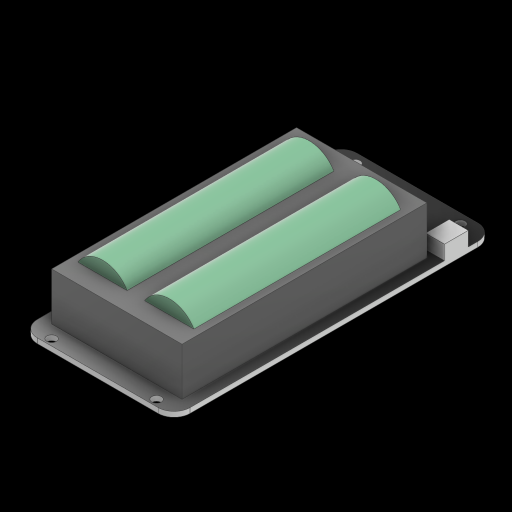
# Autodesk Inventor part: 010_Battery_2Cell
Saved by Autodesk Inventor 2024 (Build 280153000, 153)
## iProperties
Created: 2023-07-20
Part Number: 010_Battery_2Cell
Material: Generisch
Document SubType Name: Modeling
Designer: Philipp
Density: 1 g/cm^3
Appearance: Vorgabe
Author: Philipp
Autodesk Inventor part; units mm, degrees
ref_plane "YZ Plane" through (0, 0, 0) normal (1, 0, 0) x (0, 1, 0)
ref_plane "XZ Plane" through (0, 0, 0) normal (0, 1, 0) x (-1, 0, 0)
ref_plane "XY Plane" through (0, 0, 0) normal (0, 0, 1) x (1, 0, 0)
sketch "Skizze1" plane through (0, 0, 0) normal (0, 0, 1) x (1, 0, 0)
  line L0 (24, 50.25) -> (-24, 50.25)
  line L1 (-24, 50.25) -> (-24, -50.25)
  line L2 (-24, -50.25) -> (24, -50.25)
  line L3 (24, -50.25) -> (24, 50.25)
  line L4 (24, 50.25) -> (-24, -50.25) construction
  line L5 (-24, 50.25) -> (24, -50.25) construction
  point P0 (0, 0)
  dimension "d0" = 48
  dimension "d1" = 100.5
  constraints: 12 end point, 2 midpoint, 2 parallel, 1 horizontal, 1 perpendicular
  measures "d0" distance of L2.end L1.end
  measures "d1" distance of L1.end L0.end
extrude "Extrusion1" add sketch "Skizze1" along normal blind 1.6
fillet "Rundung1" radius 5 4 edges at (24, 50.25, 0.8) (-24, 50.25, 0.8) (24, -50.25, 0.8) (-24, -50.25, 0.8)
sketch "Skizze2" plane through (0, 0, 0) normal (0, 0, -1) x (-1, 0, 0)
  line L0 (-6.5, -11.25) -> (0, -11.25)
  line L1 (0, -11.25) -> (0, -17.75)
  line L2 (0, -17.75) -> (-6.5, -17.75)
  line L3 (-6.5, -17.75) -> (-6.5, -11.25)
  line L4 (-6.5, -11.25) -> (0, -17.75) construction
  line L5 (0, -11.25) -> (-6.5, -17.75) construction
  line L6 (19, -50.25) -> (-19, -50.25) projected
  line L7 (-24, -45.25) -> (-24, 45.25) projected
  point P0 (0, 0)
  point P1 (-3.25, -14.5)
  point P2 (-3.25, -17.75)
  dimension "d5" = 32.5
  dimension "d6" = 17.5
  dimension "d7" = 6.5
  dimension "d8" = 6.5
  constraints: 12 end point, 3 midpoint, 2 parallel, 1 horizontal, 1 perpendicular
  measures "d5" distance from line of L6 point (-3.25, -17.75)
  measures "d6" distance between parallel lines of L7 L3
  measures "d7" distance of L2.end L0.start
  measures "d8" distance of L0.start L0.end
extrude "Extrusion2" add sketch "Skizze2" along normal blind 5
fillet "Rundung2" radius 0.5 4 edges at (0, -11.25, -2.5) (0, -17.75, -2.5) (6.5, -17.75, -2.5) (6.5, -11.25, -2.5)
sketch "Skizze3" plane through (0, 0, 0) normal (0, 0, -1) x (-1, 0, 0)
  line L0 (17, -33.75) -> (24, -33.75)
  line L1 (24, -33.75) -> (24, -42.75)
  line L2 (24, -42.75) -> (17, -42.75)
  line L3 (17, -42.75) -> (17, -33.75)
  line L4 (17, -33.75) -> (24, -42.75) construction
  line L5 (24, -33.75) -> (17, -42.75) construction
  line L6 (19, -50.25) -> (-19, -50.25) projected
  line L7 (24, 45.25) -> (24, -45.25) projected
  point P0 (0, 0)
  point P1 (20.5, -38.25)
  dimension "d12" = 7.5
  dimension "d13" = 7
  dimension "d14" = 9
  constraints: 12 end point, 2 midpoint, 2 parallel, 1 collinear, 1 horizontal, 1 perpendicular
  measures "d12" distance between parallel lines of L6 L2
  measures "d13" distance of L1.end L2.end
  measures "d14" distance of L2.end L0.start
extrude "Extrusion3" add sketch "Skizze3" along normal blind 5
fillet "Rundung3" radius 2 2 edges at (-20.5, -33.75, -5) (-20.5, -42.75, -5)
sketch "Skizze4" plane through (0, 0, 1.6) normal (0, 0, 1) x (1, 0, 0)
  line L0 (18, 42.25) -> (24, 42.25)
  line L1 (24, 42.25) -> (24, 34.75)
  line L2 (24, 34.75) -> (18, 34.75)
  line L3 (18, 34.75) -> (18, 42.25)
  line L4 (18, 42.25) -> (24, 34.75) construction
  line L5 (24, 42.25) -> (18, 34.75) construction
  line L6 (24, -45.25) -> (24, 45.25) projected
  line L7 (-24, 45.25) -> (-24, -45.25) projected
  line L8 (19, 50.25) -> (-19, 50.25) projected
  line L9 (-22, 42.25) -> (-17.5, 42.25)
  line L10 (-17.5, 42.25) -> (-17.5, 33.25)
  line L11 (-17.5, 33.25) -> (-22, 33.25)
  line L12 (-22, 33.25) -> (-22, 42.25)
  line L13 (-22, 42.25) -> (-17.5, 33.25) construction
  line L14 (-17.5, 42.25) -> (-22, 33.25) construction
  point P0 (0, 0)
  point P1 (21, 38.5)
  point P2 (21, 42.25)
  point P3 (-19.75, 37.75)
  dimension "d19" = 8
  dimension "d20" = 7.5
  dimension "d21" = 6
  dimension "d22" = 8
  dimension "d23" = 9
  dimension "d24" = 4.5
  dimension "d25" = 2
  constraints: 24 end point, 5 midpoint, 4 parallel, 2 horizontal, 2 perpendicular, 1 collinear
  measures "d19" distance from line of L8 point (21, 42.25)
  measures "d20" distance of L2.end L0.start
  measures "d21" distance of L1.end L2.end
  measures "d22" distance between parallel lines of L8 L9
  measures "d23" distance of L9.end L10.end
  measures "d24" distance of L10.end L11.end
  measures "d25" distance between parallel lines of L7 L12
extrude "Extrusion4" add sketch "Skizze4" along normal blind 4.5
sketch "Skizze5" plane through (-22, 33.25, 1.6) normal (-1, 0, 0) x (0, 0, 1)
  line L0 (1.5, 1.5) -> (3.5, 1.5)
  line L1 (3.5, 1.5) -> (3.5, 7.5)
  line L2 (3.5, 7.5) -> (1.5, 7.5)
  line L3 (1.5, 7.5) -> (1.5, 1.5)
  line L4 (1.5, 1.5) -> (3.5, 7.5) construction
  line L5 (3.5, 1.5) -> (1.5, 7.5) construction
  line L6 (0, 9) -> (4.5, 9) projected
  line L7 (4.5, 9) -> (4.5, 0) projected
  point P0 (-1.6, -33.25)
  point P1 (2.5, 4.5)
  dimension "d28" = 1.5
  dimension "d29" = 6
  dimension "d30" = 1
  dimension "d31" = 2
  constraints: 12 end point, 2 midpoint, 2 parallel, 1 horizontal, 1 perpendicular
  measures "d28" distance between parallel lines of L6 L2
  measures "d29" distance of L0.end L1.end
  measures "d30" distance between parallel lines of L7 L1
  measures "d31" distance of L1.end L2.end
extrude "Extrusion5" add sketch "Skizze5" along normal blind 3
sketch "Skizze6" plane through (0, 0, 1.6) normal (0, 0, 1) x (1, 0, 0)
  line L0 (-20.5, 32.75) -> (20.5, 32.75)
  line L1 (20.5, 32.75) -> (20.5, -44.25)
  line L2 (20.5, -44.25) -> (-20.5, -44.25)
  line L3 (-20.5, -44.25) -> (-20.5, 32.75)
  line L4 (-20.5, 32.75) -> (20.5, -44.25) construction
  line L5 (20.5, 32.75) -> (-20.5, -44.25) construction
  line L6 (-19, -50.25) -> (19, -50.25) projected
  line L7 (24, -45.25) -> (24, 34.75) projected
  line L8 (-24, 45.25) -> (-24, -45.25) projected
  point P0 (0, 0)
  point P1 (0, -5.75)
  dimension "d34" = 6
  dimension "d35" = 3.5
  dimension "d36" = 3.5
  dimension "d37" = 77
  constraints: 12 end point, 2 midpoint, 2 parallel, 1 horizontal, 1 perpendicular
  measures "d34" distance between parallel lines of L6 L2
  measures "d35" distance between parallel lines of L7 L1
  measures "d36" distance between parallel lines of L8 L3
  measures "d37" distance of L2.end L0.start
extrude "Extrusion6" add sketch "Skizze6" along normal blind 15
sketch "Skizze7" plane through (-20.5, -44.25, 1.6) normal (0, -1, 0) x (1, 0, 0)
  circle A0 centre (10, 10.4) radius 9
  circle A1 centre (31, 10.4) radius 9
  line L0 (1.5, -1.6) -> (39.5, -1.6) projected
  line L1 (1.5, 0) -> (39.5, 0) projected
  point P0 (20.5, -1.6)
  point P1 (20.5, 0)
  dimension "d40" = 18
  dimension "d41" = 18
  dimension "d42" = 21
  dimension "d43" = 21
  dimension "d44" = 21
  dimension "d45" = 10.5
  constraints: 2 centre point, 1 midpoint
  measures "d40" diameter of A1
  measures "d41" diameter of A0
  measures "d44" distance of A1.centre A0.centre
  measures "d45" horizontal distance of point (20.5, 0) A0.centre
extrude "Extrusion7" add sketch "Skizze7" against normal blind 77
sketch "Skizze8" plane through (0, 0, 16.6) normal (0, 0, 1) x (1, 0, 0)
  line L0 (-18.2356, -44.25) -> (-18.2356, 32.75) projected
  line L1 (-18.2356, 32.75) -> (-20.5, 32.75) projected
  line L2 (-20.5, 32.75) -> (-20.5, -44.25) projected
  line L3 (-20.5, -44.25) -> (-18.2356, -44.25) projected
  line L4 (18.2356, 32.75) -> (18.2356, -44.25) projected
  line L5 (18.2356, -44.25) -> (20.5, -44.25) projected
  line L6 (20.5, -44.25) -> (20.5, 32.75) projected
  line L7 (20.5, 32.75) -> (18.2356, 32.75) projected
  line L8 (20.5, -44.25) -> (20.5, 32.75) projected
  line L9 (-20.5, 32.75) -> (20.5, 32.75)
  line L10 (20.5, 32.75) -> (20.5, 26.75)
  line L11 (20.5, 26.75) -> (-20.5, 26.75)
  line L12 (-20.5, 26.75) -> (-20.5, 32.75)
  line L13 (-20.5, -44.25) -> (20.5, -44.25)
  line L14 (20.5, -44.25) -> (20.5, -38.25)
  line L15 (20.5, -38.25) -> (-20.5, -38.25)
  line L16 (-20.5, -38.25) -> (-20.5, -44.25)
  point P0 (0, 0)
  point P1 (18.2356, -38.25)
  point P2 (-18.2356, -38.25)
  point P3 (-18.2356, 26.75)
  point P4 (18.2356, 26.75)
  dimension "d48" = 6
  dimension "d49" = 6
  constraints: 16 end point, 4 parallel, 2 horizontal, 2 perpendicular, 2 point on line
  measures "d48" distance of L9.end L10.end
  measures "d49" distance of L14.end L13.end
extrude "Extrusion8" cut sketch "Skizze8" along normal blind 10 contours L0 L15 L4 L13 | L0 L9 L4 L11
sketch "Skizze9" plane through (0, 0, 1.6) normal (0, 0, 1) x (1, 0, 0)
  line L0 (-16.5, 47.25) -> (16.5, 47.25)
  line L1 (16.5, 47.25) -> (16.5, -48.25)
  line L2 (16.5, -48.25) -> (-16.5, -48.25)
  line L3 (-16.5, -48.25) -> (-16.5, 47.25)
  line L4 (19, 50.25) -> (-19, 50.25) projected
  line L5 (20.5, 32.75) -> (-20.5, 32.75) projected
  point P0 (0, 0)
  point P1 (0, 32.75)
  point P2 (0, 47.25)
  dimension "d52" = 33
  dimension "d53" = 95.5
  dimension "d54" = 3
  dimension "d55" = 0
  constraints: 8 end point, 4 coincident, 2 midpoint, 2 parallel, 1 horizontal, 1 perpendicular
  measures "d52" distance of L0.start L0.end
  measures "d53" distance of L2.end L0.start
  measures "d54" distance between parallel lines of L4 L0
  measures "d55" horizontal distance of point (0, 32.75) point (0, 47.25)
hole "Bohrung1" at (-16.5, 47.25, 1.6) at (16.5, 47.25, 1.6) at (-16.5, -48.25, 1.6) at (16.5, -48.25, 1.6) direction (0, 0, -1) diameter 3 depth 1.6
equation "\"d45\" = 0.5 * d44"
